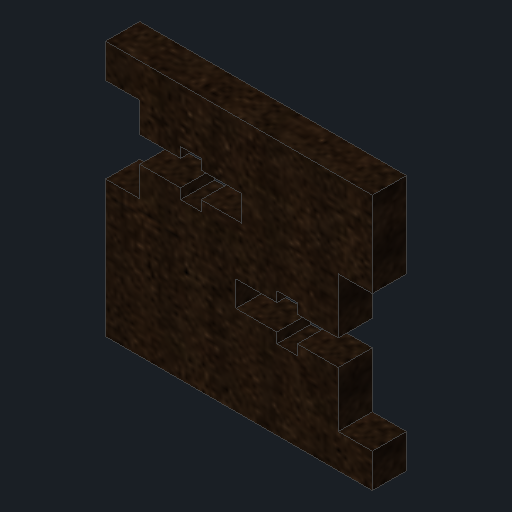
# Autodesk Inventor part: Door_LimitSwitch_Holder_Side_1
Saved by Autodesk Inventor 2024.1 (Build 281209000, 209)
## iProperties
Created: 2023-08-05
Part Number: Door_LimitSwitch_Holder_Side_1
Material: MDF Medium Density Fiberboard
Document SubType Name: Modeling
Designer: jaege
Density: 0.8 g/cm^3
Appearance: Cardboard - Corrugated
Author: jaege
Autodesk Inventor part; units mm, degrees
ref_plane "YZ Plane" through (0, 0, 0) normal (1, 0, 0) x (0, 1, 0)
ref_plane "XZ Plane" through (0, 0, 0) normal (0, 1, 0) x (-1, 0, 0)
ref_plane "XY Plane" through (0, 0, 0) normal (0, 0, 1) x (1, 0, 0)
sketch "Sketch1" plane through (0, 0, 0) normal (0, 0, 1) x (1, 0, 0)
  line L0 (-4, 10) -> (-4, 14) projected
  line L1 (0, 10) -> (-4, 10) projected
  line L2 (0, 14) -> (0, 10) construction
  line L3 (0, 14) -> (-4, 14) projected
  line L4 (-4, -16) -> (-4, 0) projected
  line L5 (0, -16) -> (-4, -16) projected
  line L6 (0, 0) -> (0, -16) construction
  line L7 (0, 0) -> (-4, 0) projected
  line L8 (0, 6.5) -> (0, 3.5) projected
  line L9 (0, 6.5) -> (12, 6.5)
  line L10 (12, 6.5) -> (12, 3.5)
  line L11 (12, 3.5) -> (0, 3.5)
  line L12 (0, 3.5) -> (0, 6.5)
  line L13 (0, 10) -> (0, 6.5)
  line L14 (0, 3.5) -> (0, 0)
  line L15 (4.8, 7.7) -> (7.2, 7.7)
  line L16 (7.2, 7.7) -> (7.2, 2.3)
  line L17 (7.2, 2.3) -> (4.8, 2.3)
  line L18 (4.8, 2.3) -> (4.8, 7.7)
  line L19 (11.3, -2.5) -> (23.3, -2.5)
  line L20 (23.3, -2.5) -> (23.3, -5.5)
  line L21 (23.3, -5.5) -> (11.3, -5.5)
  line L22 (11.3, -5.5) -> (11.3, -2.5)
  line L23 (16.1, -1.3) -> (18.5, -1.3)
  line L24 (18.5, -1.3) -> (18.5, -6.7)
  line L25 (18.5, -6.7) -> (16.1, -6.7)
  line L26 (16.1, -6.7) -> (16.1, -1.3)
  line L27 (0, 14) -> (27.3, 14)
  line L28 (27.3, 14) -> (27.3, 4)
  line L29 (27.3, 4) -> (23.3, 4)
  line L30 (23.3, 4) -> (23.3, -12)
  line L31 (23.3, -12) -> (27.3, -12)
  line L32 (27.3, -12) -> (27.3, -16)
  line L33 (27.3, -16) -> (0, -16)
  point P0 (7.2, 5)
  point P1 (12, 5)
  point P2 (6, 7.7)
  point P3 (6, 6.5)
  point P4 (16.1, -4)
  point P5 (11.3, -4)
  point P6 (17.3, -1.3)
  point P7 (17.3, -2.5)
  point P8 (23.3, -4)
  point P9 (23.3, -4)
  point P10 (4.8, 6.5)
  point P11 (7.2, 6.5)
  point P12 (7.2, 3.5)
  point P13 (4.8, 3.5)
  point P14 (18.5, -5.5)
  point P15 (16.1, -5.5)
  point P16 (16.1, -2.5)
  point P17 (18.5, -2.5)
  dimension "d0" = 12
  dimension "d1" = 3
  dimension "d2" = 5.4
  dimension "d3" = 2.4
  dimension "d4" = 12
  dimension "d5" = 3
  dimension "d6" = 2.4
  dimension "d7" = 5.4
  dimension "d8" = 4
  dimension "d10" = 10
  dimension "d11" = 23.3
  dimension "d12" = 4
  constraints: 50 end point, 10 midpoint, 9 equal length, 8 perpendicular, 6 horizontal, 2 coincident, 2 horizontal alignment, 2 point on line, 2 vertical alignment, 1 vertical
  measures "d0" distance of L10.end L11.end
  measures "d1" distance of L9.end L10.end
  measures "d2" distance of L15.end L16.end
  measures "d3" distance of L15.start L15.end
  measures "d4" distance of L20.end L21.end
  measures "d5" distance of L19.end L20.end
  measures "d6" distance of L24.end L25.end
  measures "d7" distance of L23.end L24.end
  measures "d8" distance of L28.end L29.end
  measures "d10" distance of L27.end L28.end
  measures "d11" distance between parallel lines of L30 L13
  measures "d12" distance of L31.end L32.end
extrude "Extrusion1" add sketch "Sketch1" along normal blind 4 contours L0 L3 L27 L28 L29 L30 L19 L24 L23 L26 L22 L21 L25 L31 L32 L33 L5 L4 L7 L14 L11 L18 L17 L16 L10 L9 L15 L13 L1
body "Solid1"
